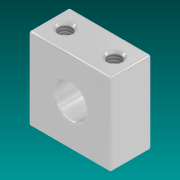
# Autodesk Inventor part: bevestegingsKoppeling axis4_5
Saved by Autodesk Inventor 2020 (Build 240168000, 168)
## iProperties
Created: 2020-05-27
Part Number: bevestegingsKoppeling axis4_5
Material: Aluminum 6061
Document SubType Name: Modeling
Designer: stefa
Density: 2.7 g/cm^3
Appearance: Aluminum - Polished
Author: stefa
Autodesk Inventor part; units mm, degrees
ref_plane "YZ Plane" through (0, 0, 0) normal (1, 0, 0) x (0, 1, 0)
ref_plane "XZ Plane" through (0, 0, 0) normal (0, 1, 0) x (-1, 0, 0)
ref_plane "XY Plane" through (0, 0, 0) normal (0, 0, 1) x (1, 0, 0)
sketch "Sketch1" plane through (0, 0, 0) normal (0, 0, 1) x (1, 0, 0)
  line L0 (-10, -10) -> (10, -10)
  line L1 (10, -10) -> (10, 10)
  line L2 (10, 10) -> (-10, 10)
  line L3 (-10, 10) -> (-10, -10)
  line L4 (-10, -10) -> (10, 10) construction
  line L5 (10, -10) -> (-10, 10) construction
  circle A0 centre (0, 0) radius 4
  dimension "d0" = 20
  dimension "d1" = 20
  dimension "d2" = 8
  constraints: 12 end point, 2 midpoint, 2 parallel, 1 centre point, 1 coincident, 1 horizontal, 1 perpendicular
  measures "d0" distance of L2.end L1.end
  measures "d1" distance of L1.end L0.end
  measures "d2" diameter of A0
extrude "Extrusion1" add sketch "Sketch1" along normal blind 10
sketch "Sketch2" plane through (-10, -10, 0) normal (0, -1, 0) x (1, 0, 0)
  line L0 (0, 0) -> (0, 10) projected
  point P0 (10, 0)
  point P1 (4, 5)
  point P2 (16, 5)
  point P3 (0, 5)
  dimension "d5" = 6
  dimension "d6" = 6
  constraints: 2 horizontal alignment, 1 midpoint
  measures "d5" horizontal distance of point (10, 0) point (4, 5)
  measures "d6" horizontal distance of point (10, 0) point (16, 5)
hole "Hole1" at (-6, -10, 5) at (6, -10, 5) direction (0, 1, 0) diameter 3.242 end through all countersink diameter 4 countersink angle 90 thread size "M4x0.7" class "6H" standard "ANSI Metric M Profile"
chamfer "Chamfer1" distance 0.5 angle 45 2 edges at (6, 10, 6.621) (-6, 10, 6.621)
fillet "Fillet2" radius 0.5 14 edges at (-4, 0, 10) (-10, 0, 10) (0, 10, 10) (10, 0, 10) (0, -10, 10) (-10, -10, 5) (10, -10, 5) (10, 10, 5) (-10, 10, 5) (-10, 0, 0) (0, 10, 0) (-4, 0, 0) (10, 0, 0) (0, -10, 0)
equation "\"d6\" = d5"
body "Solid1"
